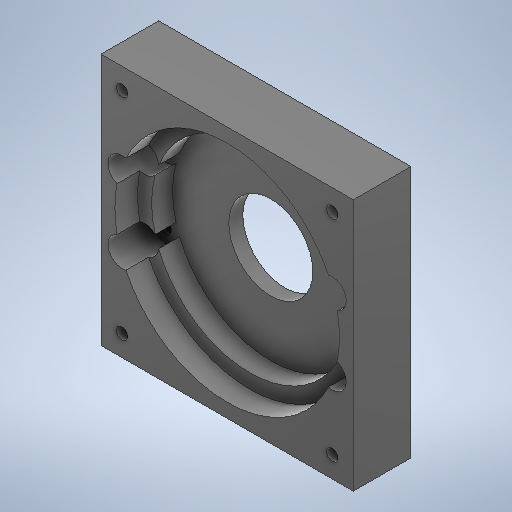
# Autodesk Inventor part: bearing_bracket1
Saved by Autodesk Inventor 2026.2 (Build 302298010, 298A)
## iProperties
Created: 2026-04-11
Part Number: bearing_bracket1
Material: ABS Plastic
Document SubType Name: Modeling
Designer: chris
Density: 1.06 g/cm^3
Appearance: Smooth - White
Author: chris
Autodesk Inventor part; units mm, degrees
ref_plane "YZ Plane" through (0, 0, 0) normal (1, 0, 0) x (0, 1, 0)
ref_plane "XZ Plane" through (0, 0, 0) normal (0, 1, 0) x (-1, 0, 0)
ref_plane "XY Plane" through (0, 0, 0) normal (0, 0, 1) x (1, 0, 0)
sketch "Sketch4" plane through (0, 0, 0) normal (0, 0, 1) x (1, 0, 0)
  line L0 (-45, -45) -> (45, -45)
  line L1 (45, -45) -> (45, 45)
  line L2 (45, 45) -> (-45, 45)
  line L3 (-45, 45) -> (-45, -45)
  line L4 (-45, -45) -> (45, 45) construction
  line L5 (45, -45) -> (-45, 45) construction
  point P0 (0, 0)
  dimension "d10" = 90
  dimension "d11" = 90
  constraints: 12 end point, 2 midpoint, 2 parallel, 1 horizontal, 1 perpendicular
  measures "d10" distance of L1.end L2.end
  measures "d11" distance of L0.end L1.end
extrude "Extrusion4" add sketch "Sketch4" along normal blind 12.47
sketch "Sketch5" plane through (0, 0, 12.47) normal (0, 0, 1) x (1, 0, 0)
  line L0 (-45, -45) -> (45, -45)
  line L1 (45, -45) -> (45, 45)
  line L2 (45, 45) -> (-45, 45)
  line L3 (-45, 45) -> (-45, -45)
  line L4 (-45, -45) -> (45, 45) construction
  line L5 (45, -45) -> (-45, 45) construction
  line L6 (45, 45) -> (-45, 45) projected
  line L7 (45, -45) -> (45, 45) projected
  circle A0 centre (0, 0) radius 40.05
  dimension "d14" = 80.1
  constraints: 12 end point, 2 collinear, 2 midpoint, 2 parallel, 1 centre point, 1 coincident, 1 horizontal, 1 perpendicular
  measures "d14" diameter of A0
extrude "Extrusion5" add sketch "Sketch5" along normal blind 8.1
sketch "Sketch6" plane through (0, 0, 12.47) normal (0, 0, 1) x (1, 0, 0)
  circle A0 centre (0, 0) radius 35
  dimension "d17" = 70
  constraints: 1 centre point, 1 coincident
  measures "d17" diameter of A0
extrude "Extrusion6" cut sketch "Sketch6" against normal through all
sketch "Sketch7" plane through (0, 0, 0) normal (0, 0, -1) x (-1, 0, 0)
  circle A0 centre (0, 0) radius 35
  circle A1 centre (0, 0) radius 35 projected
  circle A2 centre (0, 0) radius 15
  dimension "d20" = 70
  dimension "d21" = 30
  constraints: 2 centre point, 2 coincident
  measures "d20" diameter of A0
  measures "d21" diameter of A2
extrude "Extrusion7" add sketch "Sketch7" against normal blind 5
sketch "Sketch8" plane through (0, 0, 0) normal (0, 0, -1) x (-1, 0, 0)
  circle A0 centre (-37.5, -12.5) radius 2.05 projected
  circle A1 centre (-37.5, 12.5) radius 2.05 projected
  circle A2 centre (37.5, -12.5) radius 2.05 projected
  circle A3 centre (37.5, 12.5) radius 2.05 projected
  point P0 (0, 0)
hole "Hole1" at (-37.5, -12.5, 0) at (-37.5, 12.5, 0) at (37.5, -12.5, 0) at (37.5, 12.5, 0) direction (0, 0, 1) diameter 4.1 end through all
sketch "Sketch9" plane through (0, 0, 20.57) normal (0, 0, 1) x (1, 0, 0)
  arc A0 (-38.5785, -10.7566) -> (-37.3167, -14.5418) centre (-37.5, -12.5) ccw projected
  arc A1 (-37.3167, 14.5418) -> (-38.5785, 10.7566) centre (-37.5, 12.5) ccw projected
  arc A2 (38.5785, 10.7566) -> (37.3167, 14.5418) centre (37.5, 12.5) ccw projected
  arc A3 (37.3167, -14.5418) -> (38.5785, -10.7566) centre (37.5, -12.5) ccw projected
  circle A4 centre (-37.5, -12.5) radius 5
  circle A5 centre (-37.5, 12.5) radius 5
  circle A6 centre (37.5, 12.5) radius 5
  circle A7 centre (37.5, -12.5) radius 5
  point P0 (0, 0)
  dimension "d31" = 10
  dimension "d32" = 10
  dimension "d33" = 10
  dimension "d34" = 10
  constraints: 4 centre point, 4 coincident
  measures "d31" diameter of A4
  measures "d32" diameter of A5
  measures "d33" diameter of A6
  measures "d34" diameter of A7
extrude "Extrusion8" cut sketch "Sketch9" against normal blind 15.57
sketch "Sketch10" plane through (0, 0, 20.57) normal (0, 0, 1) x (1, 0, 0)
  circle A0 centre (-37.5, -37.5) radius 2.05 projected
  circle A1 centre (37.5, -37.5) radius 2.05 projected
  circle A2 centre (37.5, 37.5) radius 2.05 projected
  circle A3 centre (-37.5, 37.5) radius 2.05 projected
  circle A4 centre (37.5, -37.5) radius 2.05 projected
  circle A5 centre (-37.5, -37.5) radius 2.05 projected
  line L0 (-45, -45) -> (-45, 45) projected
  line L1 (-45, 45) -> (45, 45) projected
  line L2 (45, 45) -> (45, -45) projected
  line L3 (45, -45) -> (-45, -45) projected
  circle A6 centre (0, 0) radius 40.05 projected
  point P0 (0, 0)
hole "Hole2" at (-37.5, -37.5, 20.57) at (-37.5, 37.5, 20.57) at (37.5, 37.5, 20.57) at (37.5, -37.5, 20.57) direction (0, 0, -1) diameter 4.1 end through all
sketch "Sketch11" plane through (0, 0, 0) normal (0, 0, -1) x (-1, 0, 0)
  circle A0 centre (37.5, 37.5) radius 2.05 projected
  circle A1 centre (37.5, -37.5) radius 2.05 projected
  circle A2 centre (-37.5, -37.5) radius 2.05 projected
  circle A3 centre (-37.5, 37.5) radius 2.05 projected
  circle A4 centre (37.5, -37.5) radius 5
  circle A5 centre (-37.5, -37.5) radius 5
  circle A6 centre (-37.5, 37.5) radius 5
  circle A7 centre (37.5, 37.5) radius 5
  point P0 (0, 0)
  dimension "d44" = 10
  dimension "d45" = 10
  dimension "d46" = 10
  dimension "d47" = 10
  constraints: 4 centre point, 4 coincident
  measures "d44" diameter of A4
  measures "d45" diameter of A5
  measures "d46" diameter of A6
  measures "d47" diameter of A7
extrude "Extrusion9" cut sketch "Sketch11" against normal blind 5
body "Solid2"
